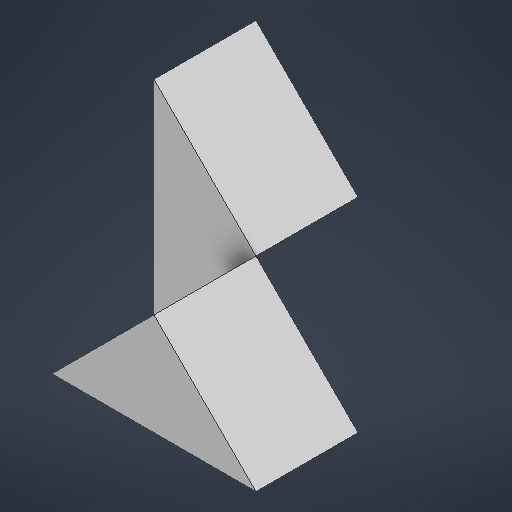
# Autodesk Inventor part: B8
Saved by Autodesk Inventor 2025.4 (Build 294407000, 407)
## iProperties
Created: 2026-05-15
Part Number: B8
Material: Generic
Document SubType Name: Modeling
Designer: VuQuan
Density: 1 g/cm^3
Appearance: Default
Author: VuQuan
Autodesk Inventor part; units mm, degrees
ref_plane "YZ Plane" through (0, 0, 0) normal (1, 0, 0) x (0, 1, 0)
ref_plane "XZ Plane" through (0, 0, 0) normal (0, 1, 0) x (-1, 0, 0)
ref_plane "XY Plane" through (0, 0, 0) normal (0, 0, 1) x (1, 0, 0)
sketch "Sketch1" plane through (0, 0, 0) normal (0, 0, 1) x (1, 0, 0)
  line L0 (-35, 0) -> (0, 35)
  line L1 (0, 35) -> (35, 0)
  line L2 (35, 0) -> (0, 0)
  line L3 (0, 0) -> (0, 35) construction
  line L4 (0, 0) -> (-35, 0)
  line L5 (0, 35) -> (-35, 70)
  line L6 (-35, 70) -> (-35, 0)
  dimension "d0" = 35
  constraints: 14 end point, 2 horizontal, 2 perpendicular, 2 vertical, 1 coincident, 1 collinear
  measures "d0" distance of L0.start L2.end
extrude "Extrusion1" add sketch "Sketch1" along normal blind 35 contours L0 L1 L2 L4
extrude "Extrusion2" add sketch "Sketch1" against normal blind 35 contours L6 L5 L0
body "Solid1"
